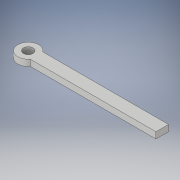
# Autodesk Inventor part: GateLid
Saved by Autodesk Inventor 2019 (Build 230136000, 136)
## iProperties
Created: 2020-12-23
Part Number: GateLid
Material: Generic
Document SubType Name: Modeling
Designer: Dell
Density: 1 g/cm^3
Appearance: Default
Author: Dell
Autodesk Inventor part; units mm, degrees
ref_plane "YZ Plane" through (0, 0, 0) normal (1, 0, 0) x (0, 1, 0)
ref_plane "XZ Plane" through (0, 0, 0) normal (0, 1, 0) x (-1, 0, 0)
ref_plane "XY Plane" through (0, 0, 0) normal (0, 0, 1) x (1, 0, 0)
sketch "Sketch1" plane through (0, 0, 0) normal (0, 1, 0) x (-1, 0, 0)
  circle A0 centre (0, 0) radius 2.3
  circle A1 centre (0, 0) radius 5
  line L0 (-4, -3) -> (-59, -3)
  line L1 (-59, -3) -> (-59, 3)
  line L2 (-59, 3) -> (-4, 3)
  line L3 (-5, 0) -> (-5, -3)
  line L4 (-5, -3) -> (-64, -3)
  line L5 (-64, -3) -> (-64, 3)
  line L6 (-64, 3) -> (-59, 3)
  dimension "d0" = 4.6
  dimension "d1" = 10
  dimension "d4" = 6
  dimension "d8" = 59
  constraints: 14 end point, 4 perpendicular, 3 point on circle, 3 point on line, 2 centre point, 2 coincident, 2 horizontal, 1 tangent
  measures "d0" diameter of A0
  measures "d1" diameter of A1
  measures "d4" distance of L0.end L1.end
  measures "d8" distance of L3.end L4.end
extrude "Extrusion2" add sketch "Sketch1" along normal blind 3
body "Solid2"
